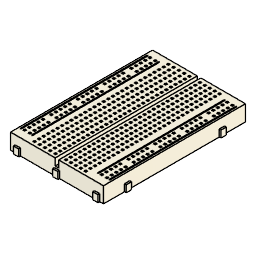
Final Robotic Car (Autodesk Fusion 360 archive; units mm, degrees)
design "Large Breadboard"
part number: 2025-09-23-22-56-39-643
part number: 2025-09-25-13-44-03-592
part number: 2025-09-25-13-51-08-297
part number: 2025-09-25-13-58-47-980
part number: 2025-09-25-14-03-45-841
Autodesk Fusion 360 part; units mm, degrees
(part 1 of 13)
sketch "Sketch1" plane through (0, 0, 0) normal (0, 0, 1) x (1, 0, 0)
  line L0 (26.5, 40.5) -> (-26.5, 40.5)
  line L1 (-26.5, 40.5) -> (-26.5, -40.5)
  line L2 (-26.5, -40.5) -> (26.5, -40.5)
  line L3 (26.5, -40.5) -> (26.5, 40.5)
  line L4 (26.5, 40.5) -> (-26.5, -40.5) construction
  line L5 (-26.5, 40.5) -> (26.5, -40.5) construction
  dimension "d1" = 81
  dimension "d2" = 53
  constraint horizontal L0
  constraint perpendicular L0 L1
  constraint parallel L0 L2
  constraint parallel L1 L3
  constraint coincident L4 origin
  constraint coincident L5 origin
  measures "d1" distance of L0.start L2.end
  measures "d2" distance of L0.start L0.end
extrude "Extrude1" add sketch "Sketch1" along normal blind 9 makes body 1
sketch "Sketch2" plane through (0, 0, 9) normal (0, 0, 1) x (-1, 0, 0)
  line L0 (-26.5, 40.5) -> (-26.5, -40.5)
  line L1 (-26.5, -40.5) -> (26.5, -40.5)
  line L2 (26.5, -40.5) -> (26.5, 40.5)
  line L3 (26.5, 40.5) -> (-26.5, 40.5)
  line L4 (-1, -41) -> (1, -41)
  line L5 (1, -41) -> (1, 41)
  line L6 (1, 41) -> (-1, 41)
  line L7 (-1, 41) -> (-1, -41)
  line L8 (-1, -41) -> (1, 41) construction
  line L9 (1, -41) -> (-1, 41) construction
  dimension "d5" = 2
  dimension "d6" = 82
  constraint horizontal L4
  constraint perpendicular L4 L5
  constraint parallel L4 L6
  constraint parallel L5 L7
  constraint coincident L8 origin
  constraint coincident L9 origin
  measures "d5" distance of L5.end L6.end
  measures "d6" distance of L4.start L6.end
extrude "Extrude2" cut sketch "Sketch2" against normal blind 4 contours L1 L3 L5 L7 bodies 1
sketch "Sketch3" plane through (0, 0, 9) normal (0, 0, 1) x (-1, 0, 0)
  line L0 (-1, -40.5) -> (-1, 40.5)
  line L1 (-1, 40.5) -> (-26.5, 40.5)
  line L2 (-26.5, 40.5) -> (-26.5, -40.5)
  line L3 (-26.5, -40.5) -> (-1, -40.5)
  line L4 (2.5, -37.5) -> (3.5, -37.5)
  line L5 (3.5, -37.5) -> (3.5, -38.5)
  line L6 (3.5, -38.5) -> (2.5, -38.5)
  line L7 (2.5, -38.5) -> (2.5, -37.5)
  line L8 (2.5, -37.5) -> (3.5, -38.5) construction
  line L9 (3.5, -37.5) -> (2.5, -38.5) construction
  line L10 (1, 40.5) -> (1, -40.5)
  line L11 (1, -40.5) -> (26.5, -40.5)
  point P0 (3, -38)
  dimension "d9" = 1
  dimension "d10" = 1
  dimension "d11" = 1.5
  dimension "d12" = 2
  constraint horizontal L4
  constraint perpendicular L4 L5
  constraint parallel L4 L6
  constraint parallel L5 L7
  constraint coincident L8 P0
  constraint coincident L9 P0
  measures "d9" distance of L5.end L6.end
  measures "d10" distance of L4.end L5.end
  measures "d11" distance of L7 L10
  measures "d12" distance of L6 L11
extrude "Extrude3" cut sketch "Sketch3" against normal blind 1 contours L4 L5 L6 L7 bodies 1
pattern_linear "R-Pattern1" count 5 spacing 3 along (-1, 0, 0) count 30 spacing 2.63 along (0, -1, 0) of "Extrude3"
sketch "Sketch4" plane through (0, 0, 9) normal (0, 0, 1) x (-1, 0, 0)
  line L0 (-1, -40.5) -> (-1, 40.5)
  line L1 (-1, 40.5) -> (-26.5, 40.5)
  line L2 (-26.5, 40.5) -> (-26.5, -40.5)
  line L3 (-26.5, -40.5) -> (-1, -40.5)
  line L4 (-3.5, -37.5) -> (-2.5, -37.5)
  line L5 (-2.5, -37.5) -> (-2.5, -38.5)
  line L6 (-2.5, -38.5) -> (-3.5, -38.5)
  line L7 (-3.5, -38.5) -> (-3.5, -37.5)
  line L8 (-3.5, -37.5) -> (-2.5, -38.5) construction
  line L9 (-2.5, -37.5) -> (-3.5, -38.5) construction
  point P0 (-3, -38)
  dimension "d19" = 1
  dimension "d20" = 1
  dimension "d21" = 2
  dimension "d22" = 1.5
  constraint horizontal L4
  constraint perpendicular L4 L5
  constraint parallel L4 L6
  constraint parallel L5 L7
  constraint coincident L8 P0
  constraint coincident L9 P0
  measures "d19" distance of L5.end L6.end
  measures "d20" distance of L4.start L6.end
  measures "d21" distance of L3 L6
  measures "d22" distance of L0 L5
extrude "Extrude4" cut sketch "Sketch4" against normal blind 1 contours L4 L5 L6 L7 bodies 1
sketch "Sketch5" plane through (0, 0, 9) normal (0, 0, 1) x (-1, 0, 0)
  line L0 (15.5, 38.77) -> (15.5, 37.77)
  line L1 (15.5, 37.77) -> (14.5, 37.77)
  line L2 (14.5, 37.77) -> (14.5, 38.77)
  line L3 (14.5, 38.77) -> (15.5, 38.77)
  line L4 (12.5, 38.77) -> (12.5, 37.77)
  line L5 (12.5, 37.77) -> (11.5, 37.77)
  line L6 (11.5, 37.77) -> (11.5, 38.77)
  line L7 (11.5, 38.77) -> (12.5, 38.77)
  line L8 (9.5, 38.77) -> (9.5, 37.77)
  line L9 (9.5, 37.77) -> (8.5, 37.77)
  line L10 (8.5, 37.77) -> (8.5, 38.77)
  line L11 (8.5, 38.77) -> (9.5, 38.77)
  line L12 (6.5, 38.77) -> (6.5, 37.77)
  line L13 (6.5, 37.77) -> (5.5, 37.77)
  line L14 (5.5, 37.77) -> (5.5, 38.77)
  line L15 (5.5, 38.77) -> (6.5, 38.77)
  line L16 (3.5, 38.77) -> (3.5, 37.77)
  line L17 (3.5, 37.77) -> (2.5, 37.77)
  line L18 (2.5, 37.77) -> (2.5, 38.77)
  line L19 (2.5, 38.77) -> (3.5, 38.77)
  line L20 (15.5, 36.14) -> (15.5, 35.14)
  line L21 (15.5, 35.14) -> (14.5, 35.14)
  line L22 (14.5, 35.14) -> (14.5, 36.14)
  line L23 (14.5, 36.14) -> (15.5, 36.14)
  line L24 (12.5, 36.14) -> (12.5, 35.14)
  line L25 (12.5, 35.14) -> (11.5, 35.14)
  line L26 (11.5, 35.14) -> (11.5, 36.14)
  line L27 (11.5, 36.14) -> (12.5, 36.14)
  line L28 (9.5, 36.14) -> (9.5, 35.14)
  line L29 (9.5, 35.14) -> (8.5, 35.14)
  line L30 (8.5, 35.14) -> (8.5, 36.14)
  line L31 (8.5, 36.14) -> (9.5, 36.14)
  line L32 (6.5, 36.14) -> (6.5, 35.14)
  line L33 (6.5, 35.14) -> (5.5, 35.14)
  line L34 (5.5, 35.14) -> (5.5, 36.14)
  line L35 (5.5, 36.14) -> (6.5, 36.14)
  line L36 (3.5, 36.14) -> (3.5, 35.14)
  line L37 (3.5, 35.14) -> (2.5, 35.14)
  line L38 (2.5, 35.14) -> (2.5, 36.14)
  line L39 (2.5, 36.14) -> (3.5, 36.14)
  line L40 (15.5, 33.51) -> (15.5, 32.51)
  line L41 (15.5, 32.51) -> (14.5, 32.51)
  line L42 (14.5, 32.51) -> (14.5, 33.51)
  line L43 (14.5, 33.51) -> (15.5, 33.51)
  line L44 (12.5, 33.51) -> (12.5, 32.51)
  line L45 (12.5, 32.51) -> (11.5, 32.51)
  line L46 (11.5, 32.51) -> (11.5, 33.51)
  line L47 (11.5, 33.51) -> (12.5, 33.51)
  line L48 (9.5, 33.51) -> (9.5, 32.51)
  line L49 (9.5, 32.51) -> (8.5, 32.51)
  line L50 (8.5, 32.51) -> (8.5, 33.51)
  line L51 (8.5, 33.51) -> (9.5, 33.51)
  line L52 (6.5, 33.51) -> (6.5, 32.51)
  line L53 (6.5, 32.51) -> (5.5, 32.51)
  line L54 (5.5, 32.51) -> (5.5, 33.51)
  line L55 (5.5, 33.51) -> (6.5, 33.51)
  line L56 (3.5, 33.51) -> (3.5, 32.51)
  line L57 (3.5, 32.51) -> (2.5, 32.51)
  line L58 (2.5, 32.51) -> (2.5, 33.51)
  line L59 (2.5, 33.51) -> (3.5, 33.51)
  line L60 (15.5, 30.88) -> (15.5, 29.88)
  line L61 (15.5, 29.88) -> (14.5, 29.88)
  line L62 (14.5, 29.88) -> (14.5, 30.88)
  line L63 (14.5, 30.88) -> (15.5, 30.88)
  line L64 (12.5, 30.88) -> (12.5, 29.88)
  line L65 (12.5, 29.88) -> (11.5, 29.88)
  line L66 (11.5, 29.88) -> (11.5, 30.88)
  line L67 (11.5, 30.88) -> (12.5, 30.88)
  line L68 (9.5, 30.88) -> (9.5, 29.88)
  line L69 (9.5, 29.88) -> (8.5, 29.88)
  line L70 (8.5, 29.88) -> (8.5, 30.88)
  line L71 (8.5, 30.88) -> (9.5, 30.88)
  line L72 (6.5, 30.88) -> (6.5, 29.88)
  line L73 (6.5, 29.88) -> (5.5, 29.88)
  line L74 (5.5, 29.88) -> (5.5, 30.88)
  line L75 (5.5, 30.88) -> (6.5, 30.88)
  line L76 (3.5, 30.88) -> (3.5, 29.88)
  line L77 (3.5, 29.88) -> (2.5, 29.88)
  line L78 (2.5, 29.88) -> (2.5, 30.88)
  line L79 (2.5, 30.88) -> (3.5, 30.88)
  line L80 (15.5, 28.25) -> (15.5, 27.25)
  line L81 (15.5, 27.25) -> (14.5, 27.25)
  line L82 (14.5, 27.25) -> (14.5, 28.25)
  line L83 (14.5, 28.25) -> (15.5, 28.25)
  line L84 (12.5, 28.25) -> (12.5, 27.25)
  line L85 (12.5, 27.25) -> (11.5, 27.25)
  line L86 (11.5, 27.25) -> (11.5, 28.25)
  line L87 (11.5, 28.25) -> (12.5, 28.25)
  line L88 (9.5, 28.25) -> (9.5, 27.25)
  line L89 (9.5, 27.25) -> (8.5, 27.25)
  line L90 (8.5, 27.25) -> (8.5, 28.25)
  line L91 (8.5, 28.25) -> (9.5, 28.25)
  line L92 (6.5, 28.25) -> (6.5, 27.25)
  line L93 (6.5, 27.25) -> (5.5, 27.25)
  line L94 (5.5, 27.25) -> (5.5, 28.25)
  line L95 (5.5, 28.25) -> (6.5, 28.25)
  line L96 (3.5, 28.25) -> (3.5, 27.25)
  line L97 (3.5, 27.25) -> (2.5, 27.25)
  line L98 (2.5, 27.25) -> (2.5, 28.25)
  line L99 (2.5, 28.25) -> (3.5, 28.25)
  line L100 (15.5, 25.62) -> (15.5, 24.62)
  line L101 (15.5, 24.62) -> (14.5, 24.62)
  line L102 (14.5, 24.62) -> (14.5, 25.62)
  line L103 (14.5, 25.62) -> (15.5, 25.62)
  line L104 (12.5, 25.62) -> (12.5, 24.62)
  line L105 (12.5, 24.62) -> (11.5, 24.62)
  line L106 (11.5, 24.62) -> (11.5, 25.62)
  line L107 (11.5, 25.62) -> (12.5, 25.62)
  line L108 (9.5, 25.62) -> (9.5, 24.62)
  line L109 (9.5, 24.62) -> (8.5, 24.62)
  line L110 (8.5, 24.62) -> (8.5, 25.62)
  line L111 (8.5, 25.62) -> (9.5, 25.62)
  line L112 (6.5, 25.62) -> (6.5, 24.62)
  line L113 (6.5, 24.62) -> (5.5, 24.62)
  line L114 (5.5, 24.62) -> (5.5, 25.62)
  line L115 (5.5, 25.62) -> (6.5, 25.62)
  line L116 (3.5, 25.62) -> (3.5, 24.62)
  line L117 (3.5, 24.62) -> (2.5, 24.62)
  line L118 (2.5, 24.62) -> (2.5, 25.62)
  line L119 (2.5, 25.62) -> (3.5, 25.62)
  line L120 (15.5, 22.99) -> (15.5, 21.99)
  line L121 (15.5, 21.99) -> (14.5, 21.99)
  line L122 (14.5, 21.99) -> (14.5, 22.99)
  line L123 (14.5, 22.99) -> (15.5, 22.99)
  line L124 (12.5, 22.99) -> (12.5, 21.99)
  line L125 (12.5, 21.99) -> (11.5, 21.99)
  line L126 (11.5, 21.99) -> (11.5, 22.99)
  line L127 (11.5, 22.99) -> (12.5, 22.99)
  line L128 (9.5, 22.99) -> (9.5, 21.99)
  line L129 (9.5, 21.99) -> (8.5, 21.99)
  line L130 (8.5, 21.99) -> (8.5, 22.99)
  line L131 (8.5, 22.99) -> (9.5, 22.99)
  line L132 (6.5, 22.99) -> (6.5, 21.99)
  line L133 (6.5, 21.99) -> (5.5, 21.99)
  line L134 (5.5, 21.99) -> (5.5, 22.99)
  line L135 (5.5, 22.99) -> (6.5, 22.99)
  line L136 (3.5, 22.99) -> (3.5, 21.99)
  line L137 (3.5, 21.99) -> (2.5, 21.99)
  line L138 (2.5, 21.99) -> (2.5, 22.99)
  line L139 (2.5, 22.99) -> (3.5, 22.99)
  line L140 (15.5, 20.36) -> (15.5, 19.36)
  line L141 (15.5, 19.36) -> (14.5, 19.36)
  line L142 (14.5, 19.36) -> (14.5, 20.36)
  line L143 (14.5, 20.36) -> (15.5, 20.36)
  line L144 (12.5, 20.36) -> (12.5, 19.36)
  line L145 (12.5, 19.36) -> (11.5, 19.36)
  line L146 (11.5, 19.36) -> (11.5, 20.36)
  line L147 (11.5, 20.36) -> (12.5, 20.36)
  line L148 (9.5, 20.36) -> (9.5, 19.36)
  line L149 (9.5, 19.36) -> (8.5, 19.36)
  line L150 (8.5, 19.36) -> (8.5, 20.36)
  line L151 (8.5, 20.36) -> (9.5, 20.36)
  line L152 (6.5, 20.36) -> (6.5, 19.36)
  line L153 (6.5, 19.36) -> (5.5, 19.36)
  line L154 (5.5, 19.36) -> (5.5, 20.36)
  line L155 (5.5, 20.36) -> (6.5, 20.36)
  line L156 (3.5, 20.36) -> (3.5, 19.36)
  line L157 (3.5, 19.36) -> (2.5, 19.36)
  line L158 (2.5, 19.36) -> (2.5, 20.36)
  line L159 (2.5, 20.36) -> (3.5, 20.36)
  line L160 (15.5, 17.73) -> (15.5, 16.73)
  line L161 (15.5, 16.73) -> (14.5, 16.73)
  line L162 (14.5, 16.73) -> (14.5, 17.73)
  line L163 (14.5, 17.73) -> (15.5, 17.73)
  line L164 (12.5, 17.73) -> (12.5, 16.73)
  line L165 (12.5, 16.73) -> (11.5, 16.73)
  line L166 (11.5, 16.73) -> (11.5, 17.73)
  line L167 (11.5, 17.73) -> (12.5, 17.73)
  line L168 (9.5, 17.73) -> (9.5, 16.73)
  line L169 (9.5, 16.73) -> (8.5, 16.73)
  line L170 (8.5, 16.73) -> (8.5, 17.73)
  line L171 (8.5, 17.73) -> (9.5, 17.73)
  line L172 (6.5, 17.73) -> (6.5, 16.73)
  line L173 (6.5, 16.73) -> (5.5, 16.73)
  line L174 (5.5, 16.73) -> (5.5, 17.73)
  line L175 (5.5, 17.73) -> (6.5, 17.73)
  line L176 (3.5, 17.73) -> (3.5, 16.73)
  line L177 (3.5, 16.73) -> (2.5, 16.73)
  line L178 (2.5, 16.73) -> (2.5, 17.73)
  line L179 (2.5, 17.73) -> (3.5, 17.73)
  line L180 (15.5, 15.1) -> (15.5, 14.1)
  line L181 (15.5, 14.1) -> (14.5, 14.1)
  line L182 (14.5, 14.1) -> (14.5, 15.1)
  line L183 (14.5, 15.1) -> (15.5, 15.1)
  line L184 (12.5, 15.1) -> (12.5, 14.1)
  line L185 (12.5, 14.1) -> (11.5, 14.1)
  line L186 (11.5, 14.1) -> (11.5, 15.1)
  line L187 (11.5, 15.1) -> (12.5, 15.1)
  line L188 (9.5, 15.1) -> (9.5, 14.1)
  line L189 (9.5, 14.1) -> (8.5, 14.1)
  line L190 (8.5, 14.1) -> (8.5, 15.1)
  line L191 (8.5, 15.1) -> (9.5, 15.1)
  line L192 (6.5, 15.1) -> (6.5, 14.1)
  line L193 (6.5, 14.1) -> (5.5, 14.1)
  line L194 (5.5, 14.1) -> (5.5, 15.1)
  line L195 (5.5, 15.1) -> (6.5, 15.1)
  line L196 (3.5, 15.1) -> (3.5, 14.1)
  line L197 (3.5, 14.1) -> (2.5, 14.1)
  line L198 (2.5, 14.1) -> (2.5, 15.1)
  line L199 (2.5, 15.1) -> (3.5, 15.1)
  line L200 (15.5, 12.47) -> (15.5, 11.47)
  line L201 (15.5, 11.47) -> (14.5, 11.47)
  line L202 (14.5, 11.47) -> (14.5, 12.47)
  line L203 (14.5, 12.47) -> (15.5, 12.47)
  line L204 (12.5, 12.47) -> (12.5, 11.47)
  line L205 (12.5, 11.47) -> (11.5, 11.47)
  line L206 (11.5, 11.47) -> (11.5, 12.47)
  line L207 (11.5, 12.47) -> (12.5, 12.47)
  line L208 (9.5, 12.47) -> (9.5, 11.47)
  line L209 (9.5, 11.47) -> (8.5, 11.47)
  line L210 (8.5, 11.47) -> (8.5, 12.47)
  line L211 (8.5, 12.47) -> (9.5, 12.47)
  line L212 (6.5, 12.47) -> (6.5, 11.47)
  line L213 (6.5, 11.47) -> (5.5, 11.47)
  line L214 (5.5, 11.47) -> (5.5, 12.47)
  line L215 (5.5, 12.47) -> (6.5, 12.47)
  line L216 (3.5, 12.47) -> (3.5, 11.47)
  line L217 (3.5, 11.47) -> (2.5, 11.47)
  line L218 (2.5, 11.47) -> (2.5, 12.47)
  line L219 (2.5, 12.47) -> (3.5, 12.47)
  line L220 (15.5, 9.84) -> (15.5, 8.84)
  line L221 (15.5, 8.84) -> (14.5, 8.84)
  line L222 (14.5, 8.84) -> (14.5, 9.84)
  line L223 (14.5, 9.84) -> (15.5, 9.84)
  line L224 (12.5, 9.84) -> (12.5, 8.84)
  line L225 (12.5, 8.84) -> (11.5, 8.84)
  line L226 (11.5, 8.84) -> (11.5, 9.84)
  line L227 (11.5, 9.84) -> (12.5, 9.84)
  line L228 (9.5, 9.84) -> (9.5, 8.84)
  line L229 (9.5, 8.84) -> (8.5, 8.84)
  line L230 (8.5, 8.84) -> (8.5, 9.84)
  line L231 (8.5, 9.84) -> (9.5, 9.84)
  line L232 (6.5, 9.84) -> (6.5, 8.84)
  line L233 (6.5, 8.84) -> (5.5, 8.84)
  line L234 (5.5, 8.84) -> (5.5, 9.84)
  line L235 (5.5, 9.84) -> (6.5, 9.84)
  line L236 (3.5, 9.84) -> (3.5, 8.84)
  line L237 (3.5, 8.84) -> (2.5, 8.84)
  line L238 (2.5, 8.84) -> (2.5, 9.84)
  line L239 (2.5, 9.84) -> (3.5, 9.84)
  line L240 (15.5, 7.21) -> (15.5, 6.21)
  line L241 (15.5, 6.21) -> (14.5, 6.21)
  line L242 (14.5, 6.21) -> (14.5, 7.21)
  line L243 (14.5, 7.21) -> (15.5, 7.21)
  line L244 (12.5, 7.21) -> (12.5, 6.21)
  line L245 (12.5, 6.21) -> (11.5, 6.21)
  line L246 (11.5, 6.21) -> (11.5, 7.21)
  line L247 (11.5, 7.21) -> (12.5, 7.21)
  line L248 (9.5, 7.21) -> (9.5, 6.21)
  line L249 (9.5, 6.21) -> (8.5, 6.21)
  line L250 (8.5, 6.21) -> (8.5, 7.21)
  line L251 (8.5, 7.21) -> (9.5, 7.21)
  line L252 (6.5, 7.21) -> (6.5, 6.21)
  line L253 (6.5, 6.21) -> (5.5, 6.21)
  line L254 (5.5, 6.21) -> (5.5, 7.21)
  line L255 (5.5, 7.21) -> (6.5, 7.21)
  line L256 (3.5, 7.21) -> (3.5, 6.21)
  line L257 (3.5, 6.21) -> (2.5, 6.21)
  line L258 (2.5, 6.21) -> (2.5, 7.21)
  line L259 (2.5, 7.21) -> (3.5, 7.21)
  line L260 (15.5, 4.58) -> (15.5, 3.58)
  line L261 (15.5, 3.58) -> (14.5, 3.58)
  line L262 (14.5, 3.58) -> (14.5, 4.58)
  line L263 (14.5, 4.58) -> (15.5, 4.58)
  line L264 (12.5, 4.58) -> (12.5, 3.58)
  line L265 (12.5, 3.58) -> (11.5, 3.58)
  line L266 (11.5, 3.58) -> (11.5, 4.58)
  line L267 (11.5, 4.58) -> (12.5, 4.58)
  line L268 (9.5, 4.58) -> (9.5, 3.58)
  line L269 (9.5, 3.58) -> (8.5, 3.58)
  line L270 (8.5, 3.58) -> (8.5, 4.58)
  line L271 (8.5, 4.58) -> (9.5, 4.58)
  line L272 (6.5, 4.58) -> (6.5, 3.58)
  line L273 (6.5, 3.58) -> (5.5, 3.58)
  line L274 (5.5, 3.58) -> (5.5, 4.58)
  line L275 (5.5, 4.58) -> (6.5, 4.58)
  line L276 (3.5, 4.58) -> (3.5, 3.58)
  line L277 (3.5, 3.58) -> (2.5, 3.58)
  line L278 (2.5, 3.58) -> (2.5, 4.58)
  line L279 (2.5, 4.58) -> (3.5, 4.58)
  line L280 (15.5, 1.95) -> (15.5, 0.95)
  line L281 (15.5, 0.95) -> (14.5, 0.95)
  line L282 (14.5, 0.95) -> (14.5, 1.95)
  line L283 (14.5, 1.95) -> (15.5, 1.95)
  line L284 (12.5, 1.95) -> (12.5, 0.95)
  line L285 (12.5, 0.95) -> (11.5, 0.95)
  line L286 (11.5, 0.95) -> (11.5, 1.95)
  line L287 (11.5, 1.95) -> (12.5, 1.95)
  line L288 (9.5, 1.95) -> (9.5, 0.95)
  line L289 (9.5, 0.95) -> (8.5, 0.95)
  line L290 (8.5, 0.95) -> (8.5, 1.95)
  line L291 (8.5, 1.95) -> (9.5, 1.95)
  line L292 (6.5, 1.95) -> (6.5, 0.95)
  line L293 (6.5, 0.95) -> (5.5, 0.95)
  line L294 (5.5, 0.95) -> (5.5, 1.95)
  line L295 (5.5, 1.95) -> (6.5, 1.95)
  line L296 (3.5, 1.95) -> (3.5, 0.95)
  line L297 (3.5, 0.95) -> (2.5, 0.95)
  line L298 (2.5, 0.95) -> (2.5, 1.95)
  line L299 (2.5, 1.95) -> (3.5, 1.95)
  line L300 (15.5, -0.68) -> (15.5, -1.68)
  line L301 (15.5, -1.68) -> (14.5, -1.68)
  line L302 (14.5, -1.68) -> (14.5, -0.68)
  line L303 (14.5, -0.68) -> (15.5, -0.68)
  line L304 (12.5, -0.68) -> (12.5, -1.68)
  line L305 (12.5, -1.68) -> (11.5, -1.68)
  line L306 (11.5, -1.68) -> (11.5, -0.68)
  line L307 (11.5, -0.68) -> (12.5, -0.68)
  line L308 (9.5, -0.68) -> (9.5, -1.68)
  line L309 (9.5, -1.68) -> (8.5, -1.68)
  line L310 (8.5, -1.68) -> (8.5, -0.68)
  line L311 (8.5, -0.68) -> (9.5, -0.68)
  line L312 (6.5, -0.68) -> (6.5, -1.68)
  line L313 (6.5, -1.68) -> (5.5, -1.68)
  line L314 (5.5, -1.68) -> (5.5, -0.68)
  line L315 (5.5, -0.68) -> (6.5, -0.68)
  line L316 (3.5, -0.68) -> (3.5, -1.68)
  line L317 (3.5, -1.68) -> (2.5, -1.68)
  line L318 (2.5, -1.68) -> (2.5, -0.68)
  line L319 (2.5, -0.68) -> (3.5, -0.68)
  line L320 (15.5, -3.31) -> (15.5, -4.31)
  line L321 (15.5, -4.31) -> (14.5, -4.31)
  line L322 (14.5, -4.31) -> (14.5, -3.31)
  line L323 (14.5, -3.31) -> (15.5, -3.31)
  line L324 (12.5, -3.31) -> (12.5, -4.31)
  line L325 (12.5, -4.31) -> (11.5, -4.31)
  line L326 (11.5, -4.31) -> (11.5, -3.31)
  line L327 (11.5, -3.31) -> (12.5, -3.31)
  line L328 (9.5, -3.31) -> (9.5, -4.31)
  line L329 (9.5, -4.31) -> (8.5, -4.31)
  line L330 (8.5, -4.31) -> (8.5, -3.31)
  line L331 (8.5, -3.31) -> (9.5, -3.31)
  line L332 (6.5, -3.31) -> (6.5, -4.31)
  line L333 (6.5, -4.31) -> (5.5, -4.31)
  line L334 (5.5, -4.31) -> (5.5, -3.31)
  line L335 (5.5, -3.31) -> (6.5, -3.31)
  line L336 (3.5, -3.31) -> (3.5, -4.31)
  line L337 (3.5, -4.31) -> (2.5, -4.31)
  line L338 (2.5, -4.31) -> (2.5, -3.31)
  line L339 (2.5, -3.31) -> (3.5, -3.31)
  line L340 (15.5, -5.94) -> (15.5, -6.94)
  line L341 (15.5, -6.94) -> (14.5, -6.94)
  line L342 (14.5, -6.94) -> (14.5, -5.94)
  line L343 (14.5, -5.94) -> (15.5, -5.94)
  line L344 (12.5, -5.94) -> (12.5, -6.94)
  line L345 (12.5, -6.94) -> (11.5, -6.94)
  line L346 (11.5, -6.94) -> (11.5, -5.94)
  line L347 (11.5, -5.94) -> (12.5, -5.94)
  line L348 (9.5, -5.94) -> (9.5, -6.94)
  line L349 (9.5, -6.94) -> (8.5, -6.94)
  line L350 (8.5, -6.94) -> (8.5, -5.94)
  line L351 (8.5, -5.94) -> (9.5, -5.94)
  line L352 (6.5, -5.94) -> (6.5, -6.94)
  line L353 (6.5, -6.94) -> (5.5, -6.94)
  line L354 (5.5, -6.94) -> (5.5, -5.94)
  line L355 (5.5, -5.94) -> (6.5, -5.94)
  line L356 (3.5, -5.94) -> (3.5, -6.94)
  line L357 (3.5, -6.94) -> (2.5, -6.94)
  line L358 (2.5, -6.94) -> (2.5, -5.94)
  line L359 (2.5, -5.94) -> (3.5, -5.94)
  line L360 (15.5, -8.57) -> (15.5, -9.57)
  line L361 (15.5, -9.57) -> (14.5, -9.57)
  line L362 (14.5, -9.57) -> (14.5, -8.57)
  line L363 (14.5, -8.57) -> (15.5, -8.57)
  line L364 (12.5, -8.57) -> (12.5, -9.57)
  line L365 (12.5, -9.57) -> (11.5, -9.57)
  line L366 (11.5, -9.57) -> (11.5, -8.57)
  line L367 (11.5, -8.57) -> (12.5, -8.57)
  line L368 (9.5, -8.57) -> (9.5, -9.57)
  line L369 (9.5, -9.57) -> (8.5, -9.57)
  line L370 (8.5, -9.57) -> (8.5, -8.57)
  line L371 (8.5, -8.57) -> (9.5, -8.57)
  line L372 (6.5, -8.57) -> (6.5, -9.57)
  line L373 (6.5, -9.57) -> (5.5, -9.57)
  line L374 (5.5, -9.57) -> (5.5, -8.57)
  line L375 (5.5, -8.57) -> (6.5, -8.57)
  line L376 (3.5, -8.57) -> (3.5, -9.57)
  line L377 (3.5, -9.57) -> (2.5, -9.57)
  line L378 (2.5, -9.57) -> (2.5, -8.57)
  line L379 (2.5, -8.57) -> (3.5, -8.57)
  line L380 (15.5, -11.2) -> (15.5, -12.2)
  line L381 (15.5, -12.2) -> (14.5, -12.2)
  line L382 (14.5, -12.2) -> (14.5, -11.2)
  line L383 (14.5, -11.2) -> (15.5, -11.2)
  line L384 (12.5, -11.2) -> (12.5, -12.2)
  line L385 (12.5, -12.2) -> (11.5, -12.2)
  line L386 (11.5, -12.2) -> (11.5, -11.2)
  line L387 (11.5, -11.2) -> (12.5, -11.2)
  line L388 (9.5, -11.2) -> (9.5, -12.2)
  line L389 (9.5, -12.2) -> (8.5, -12.2)
  line L390 (8.5, -12.2) -> (8.5, -11.2)
  line L391 (8.5, -11.2) -> (9.5, -11.2)
  line L392 (6.5, -11.2) -> (6.5, -12.2)
  line L393 (6.5, -12.2) -> (5.5, -12.2)
  line L394 (5.5, -12.2) -> (5.5, -11.2)
  line L395 (5.5, -11.2) -> (6.5, -11.2)
  line L396 (3.5, -11.2) -> (3.5, -12.2)
  line L397 (3.5, -12.2) -> (2.5, -12.2)
  line L398 (2.5, -12.2) -> (2.5, -11.2)
  line L399 (2.5, -11.2) -> (3.5, -11.2)
  line L400 (15.5, -13.83) -> (15.5, -14.83)
  line L401 (15.5, -14.83) -> (14.5, -14.83)
  line L402 (14.5, -14.83) -> (14.5, -13.83)
  line L403 (14.5, -13.83) -> (15.5, -13.83)
  line L404 (12.5, -13.83) -> (12.5, -14.83)
  line L405 (12.5, -14.83) -> (11.5, -14.83)
  line L406 (11.5, -14.83) -> (11.5, -13.83)
  line L407 (11.5, -13.83) -> (12.5, -13.83)
  line L408 (9.5, -13.83) -> (9.5, -14.83)
  line L409 (9.5, -14.83) -> (8.5, -14.83)
  line L410 (8.5, -14.83) -> (8.5, -13.83)
  line L411 (8.5, -13.83) -> (9.5, -13.83)
  line L412 (6.5, -13.83) -> (6.5, -14.83)
  line L413 (6.5, -14.83) -> (5.5, -14.83)
  line L414 (5.5, -14.83) -> (5.5, -13.83)
  line L415 (5.5, -13.83) -> (6.5, -13.83)
  line L416 (3.5, -13.83) -> (3.5, -14.83)
  line L417 (3.5, -14.83) -> (2.5, -14.83)
  line L418 (2.5, -14.83) -> (2.5, -13.83)
  line L419 (2.5, -13.83) -> (3.5, -13.83)
  line L420 (15.5, -16.46) -> (15.5, -17.46)
  line L421 (15.5, -17.46) -> (14.5, -17.46)
  line L422 (14.5, -17.46) -> (14.5, -16.46)
  line L423 (14.5, -16.46) -> (15.5, -16.46)
  line L424 (12.5, -16.46) -> (12.5, -17.46)
  line L425 (12.5, -17.46) -> (11.5, -17.46)
  line L426 (11.5, -17.46) -> (11.5, -16.46)
  line L427 (11.5, -16.46) -> (12.5, -16.46)
  line L428 (9.5, -16.46) -> (9.5, -17.46)
  line L429 (9.5, -17.46) -> (8.5, -17.46)
  line L430 (8.5, -17.46) -> (8.5, -16.46)
  line L431 (8.5, -16.46) -> (9.5, -16.46)
  line L432 (6.5, -16.46) -> (6.5, -17.46)
  line L433 (6.5, -17.46) -> (5.5, -17.46)
  line L434 (5.5, -17.46) -> (5.5, -16.46)
  line L435 (5.5, -16.46) -> (6.5, -16.46)
  line L436 (3.5, -16.46) -> (3.5, -17.46)
  line L437 (3.5, -17.46) -> (2.5, -17.46)
  line L438 (2.5, -17.46) -> (2.5, -16.46)
  line L439 (2.5, -16.46) -> (3.5, -16.46)
  line L440 (15.5, -19.09) -> (15.5, -20.09)
  line L441 (15.5, -20.09) -> (14.5, -20.09)
  line L442 (14.5, -20.09) -> (14.5, -19.09)
  line L443 (14.5, -19.09) -> (15.5, -19.09)
  line L444 (12.5, -19.09) -> (12.5, -20.09)
  line L445 (12.5, -20.09) -> (11.5, -20.09)
  line L446 (11.5, -20.09) -> (11.5, -19.09)
  line L447 (11.5, -19.09) -> (12.5, -19.09)
  line L448 (9.5, -19.09) -> (9.5, -20.09)
  line L449 (9.5, -20.09) -> (8.5, -20.09)
  line L450 (8.5, -20.09) -> (8.5, -19.09)
  line L451 (8.5, -19.09) -> (9.5, -19.09)
  line L452 (6.5, -19.09) -> (6.5, -20.09)
  line L453 (6.5, -20.09) -> (5.5, -20.09)
  line L454 (5.5, -20.09) -> (5.5, -19.09)
  line L455 (5.5, -19.09) -> (6.5, -19.09)
  line L456 (3.5, -19.09) -> (3.5, -20.09)
  line L457 (3.5, -20.09) -> (2.5, -20.09)
  line L458 (2.5, -20.09) -> (2.5, -19.09)
  line L459 (2.5, -19.09) -> (3.5, -19.09)
  line L460 (15.5, -21.72) -> (15.5, -22.72)
  line L461 (15.5, -22.72) -> (14.5, -22.72)
  line L462 (14.5, -22.72) -> (14.5, -21.72)
  line L463 (14.5, -21.72) -> (15.5, -21.72)
  line L464 (12.5, -21.72) -> (12.5, -22.72)
  line L465 (12.5, -22.72) -> (11.5, -22.72)
  line L466 (11.5, -22.72) -> (11.5, -21.72)
  line L467 (11.5, -21.72) -> (12.5, -21.72)
  line L468 (9.5, -21.72) -> (9.5, -22.72)
  line L469 (9.5, -22.72) -> (8.5, -22.72)
  line L470 (8.5, -22.72) -> (8.5, -21.72)
  line L471 (8.5, -21.72) -> (9.5, -21.72)
  line L472 (6.5, -21.72) -> (6.5, -22.72)
  line L473 (6.5, -22.72) -> (5.5, -22.72)
  line L474 (5.5, -22.72) -> (5.5, -21.72)
  line L475 (5.5, -21.72) -> (6.5, -21.72)
  line L476 (3.5, -21.72) -> (3.5, -22.72)
  line L477 (3.5, -22.72) -> (2.5, -22.72)
  line L478 (2.5, -22.72) -> (2.5, -21.72)
  line L479 (2.5, -21.72) -> (3.5, -21.72)
  line L480 (15.5, -24.35) -> (15.5, -25.35)
  line L481 (15.5, -25.35) -> (14.5, -25.35)
  line L482 (14.5, -25.35) -> (14.5, -24.35)
  line L483 (14.5, -24.35) -> (15.5, -24.35)
  line L484 (12.5, -24.35) -> (12.5, -25.35)
  line L485 (12.5, -25.35) -> (11.5, -25.35)
  line L486 (11.5, -25.35) -> (11.5, -24.35)
  line L487 (11.5, -24.35) -> (12.5, -24.35)
  line L488 (9.5, -24.35) -> (9.5, -25.35)
  line L489 (9.5, -25.35) -> (8.5, -25.35)
  line L490 (8.5, -25.35) -> (8.5, -24.35)
  line L491 (8.5, -24.35) -> (9.5, -24.35)
  line L492 (6.5, -24.35) -> (6.5, -25.35)
  line L493 (6.5, -25.35) -> (5.5, -25.35)
  line L494 (5.5, -25.35) -> (5.5, -24.35)
  line L495 (5.5, -24.35) -> (6.5, -24.35)
  line L496 (3.5, -24.35) -> (3.5, -25.35)
  line L497 (3.5, -25.35) -> (2.5, -25.35)
  line L498 (2.5, -25.35) -> (2.5, -24.35)
  line L499 (2.5, -24.35) -> (3.5, -24.35)
  line L500 (15.5, -26.98) -> (15.5, -27.98)
  line L501 (15.5, -27.98) -> (14.5, -27.98)
  line L502 (14.5, -27.98) -> (14.5, -26.98)
  line L503 (14.5, -26.98) -> (15.5, -26.98)
  line L504 (12.5, -26.98) -> (12.5, -27.98)
  line L505 (12.5, -27.98) -> (11.5, -27.98)
  line L506 (11.5, -27.98) -> (11.5, -26.98)
  line L507 (11.5, -26.98) -> (12.5, -26.98)
  line L508 (9.5, -26.98) -> (9.5, -27.98)
  line L509 (9.5, -27.98) -> (8.5, -27.98)
  line L510 (8.5, -27.98) -> (8.5, -26.98)
  line L511 (8.5, -26.98) -> (9.5, -26.98)
  line L512 (6.5, -26.98) -> (6.5, -27.98)
  line L513 (6.5, -27.98) -> (5.5, -27.98)
  line L514 (5.5, -27.98) -> (5.5, -26.98)
  line L515 (5.5, -26.98) -> (6.5, -26.98)
  line L516 (3.5, -26.98) -> (3.5, -27.98)
  line L517 (3.5, -27.98) -> (2.5, -27.98)
  line L518 (2.5, -27.98) -> (2.5, -26.98)
  line L519 (2.5, -26.98) -> (3.5, -26.98)
  line L520 (15.5, -29.61) -> (15.5, -30.61)
  line L521 (15.5, -30.61) -> (14.5, -30.61)
  line L522 (14.5, -30.61) -> (14.5, -29.61)
  line L523 (14.5, -29.61) -> (15.5, -29.61)
  line L524 (12.5, -29.61) -> (12.5, -30.61)
  line L525 (12.5, -30.61) -> (11.5, -30.61)
  line L526 (11.5, -30.61) -> (11.5, -29.61)
  line L527 (11.5, -29.61) -> (12.5, -29.61)
  line L528 (9.5, -29.61) -> (9.5, -30.61)
  line L529 (9.5, -30.61) -> (8.5, -30.61)
  line L530 (8.5, -30.61) -> (8.5, -29.61)
  line L531 (8.5, -29.61) -> (9.5, -29.61)
  line L532 (6.5, -29.61) -> (6.5, -30.61)
  line L533 (6.5, -30.61) -> (5.5, -30.61)
  line L534 (5.5, -30.61) -> (5.5, -29.61)
  line L535 (5.5, -29.61) -> (6.5, -29.61)
  line L536 (3.5, -29.61) -> (3.5, -30.61)
  line L537 (3.5, -30.61) -> (2.5, -30.61)
  line L538 (2.5, -30.61) -> (2.5, -29.61)
  line L539 (2.5, -29.61) -> (3.5, -29.61)
  line L540 (15.5, -32.24) -> (15.5, -33.24)
  line L541 (15.5, -33.24) -> (14.5, -33.24)
  line L542 (14.5, -33.24) -> (14.5, -32.24)
  line L543 (14.5, -32.24) -> (15.5, -32.24)
  line L544 (12.5, -32.24) -> (12.5, -33.24)
  line L545 (12.5, -33.24) -> (11.5, -33.24)
  line L546 (11.5, -33.24) -> (11.5, -32.24)
  line L547 (11.5, -32.24) -> (12.5, -32.24)
  line L548 (9.5, -32.24) -> (9.5, -33.24)
  line L549 (9.5, -33.24) -> (8.5, -33.24)
  line L550 (8.5, -33.24) -> (8.5, -32.24)
  line L551 (8.5, -32.24) -> (9.5, -32.24)
  line L552 (6.5, -32.24) -> (6.5, -33.24)
  line L553 (6.5, -33.24) -> (5.5, -33.24)
  line L554 (5.5, -33.24) -> (5.5, -32.24)
  line L555 (5.5, -32.24) -> (6.5, -32.24)
  line L556 (3.5, -32.24) -> (3.5, -33.24)
  line L557 (3.5, -33.24) -> (2.5, -33.24)
  line L558 (2.5, -33.24) -> (2.5, -32.24)
  line L559 (2.5, -32.24) -> (3.5, -32.24)
  line L560 (15.5, -34.87) -> (15.5, -35.87)
  line L561 (15.5, -35.87) -> (14.5, -35.87)
  line L562 (14.5, -35.87) -> (14.5, -34.87)
  line L563 (14.5, -34.87) -> (15.5, -34.87)
  line L564 (12.5, -34.87) -> (12.5, -35.87)
  line L565 (12.5, -35.87) -> (11.5, -35.87)
  line L566 (11.5, -35.87) -> (11.5, -34.87)
  line L567 (11.5, -34.87) -> (12.5, -34.87)
  line L568 (9.5, -34.87) -> (9.5, -35.87)
  line L569 (9.5, -35.87) -> (8.5, -35.87)
  line L570 (8.5, -35.87) -> (8.5, -34.87)
  line L571 (8.5, -34.87) -> (9.5, -34.87)
  line L572 (6.5, -34.87) -> (6.5, -35.87)
  line L573 (6.5, -35.87) -> (5.5, -35.87)
  line L574 (5.5, -35.87) -> (5.5, -34.87)
  line L575 (5.5, -34.87) -> (6.5, -34.87)
  line L576 (3.5, -34.87) -> (3.5, -35.87)
  line L577 (3.5, -35.87) -> (2.5, -35.87)
  line L578 (2.5, -35.87) -> (2.5, -34.87)
  line L579 (2.5, -34.87) -> (3.5, -34.87)
  line L580 (15.5, -37.5) -> (15.5, -38.5)
  line L581 (15.5, -38.5) -> (14.5, -38.5)
  line L582 (14.5, -38.5) -> (14.5, -37.5)
  line L583 (14.5, -37.5) -> (15.5, -37.5)
  line L584 (12.5, -37.5) -> (12.5, -38.5)
  line L585 (12.5, -38.5) -> (11.5, -38.5)
  line L586 (11.5, -38.5) -> (11.5, -37.5)
  line L587 (11.5, -37.5) -> (12.5, -37.5)
  line L588 (9.5, -37.5) -> (9.5, -38.5)
  line L589 (9.5, -38.5) -> (8.5, -38.5)
  line L590 (8.5, -38.5) -> (8.5, -37.5)
  line L591 (8.5, -37.5) -> (9.5, -37.5)
  line L592 (6.5, -37.5) -> (6.5, -38.5)
  line L593 (6.5, -38.5) -> (5.5, -38.5)
  line L594 (5.5, -38.5) -> (5.5, -37.5)
  line L595 (5.5, -37.5) -> (6.5, -37.5)
  line L596 (3.5, -37.5) -> (3.5, -38.5)
  line L597 (3.5, -38.5) -> (2.5, -38.5)
  line L598 (2.5, -38.5) -> (2.5, -37.5)
  line L599 (2.5, -37.5) -> (3.5, -37.5)
  line L600 (1, 40.5) -> (1, -40.5)
  line L601 (1, -40.5) -> (26.5, -40.5)
  line L602 (26.5, -40.5) -> (26.5, 40.5)
  line L603 (26.5, 40.5) -> (1, 40.5)
pattern_linear "R-Pattern2" count 30 spacing 2.63 along (0, -1, 0) count 5 spacing 2.8 along (1, 0, 0) of "Extrude4"
sketch "Sketch9" plane through (0, -40.5, 0) normal (0, -1, 0) x (1, 0, 0)
  line L0 (1, 9) -> (1, 5)
  line L1 (1, 5) -> (-1, 5)
  line L2 (-1, 5) -> (-1, 9)
  line L3 (-1, 9) -> (-26.5, 9)
  line L4 (-26.5, 9) -> (-26.5, 0)
  line L5 (-26.5, 0) -> (26.5, 0)
  line L6 (26.5, 0) -> (26.5, 9)
  line L7 (26.5, 9) -> (1, 9)
  line L8 (-20.8174, 4) -> (-23.8174, 4)
  line L9 (-23.8174, 4) -> (-23.8174, -4)
  line L10 (-23.8174, -4) -> (-20.8174, -4)
  line L11 (-20.8174, -4) -> (-20.8174, 4)
  line L12 (-20.8174, 4) -> (-23.8174, -4) construction
  line L13 (-23.8174, 4) -> (-20.8174, -4) construction
  point P0 (-22.3174, 0)
  dimension "d35" = 3
  dimension "d36" = 8
  constraint horizontal L8
  constraint perpendicular L8 L9
  constraint parallel L8 L10
  constraint parallel L9 L11
  constraint coincident L12 P0
  constraint coincident L13 P0
  constraint coincident L5 P0
  measures "d35" distance of L9.end L10.end
  measures "d36" distance of L8.start L10.end
extrude "Extrude6" add sketch "Sketch9" along normal blind 1 contours L5 L8 L9 L11 bodies 1
extrude "Extrude7" add 1 faces at (-21.8174, -41.5, 1.3333) along direction (0, 1, 0) blind 83 on bodies 1 bodies 1
extrude "Extrude8" cut 1 faces at (-21.8174, 41.5, 1.3333) along direction (0, -1, 0) blind 2 on bodies 1 bodies 1
sketch "Sketch10" plane through (0, -40.5, 0) normal (0, -1, 0) x (1, 0, 0)
  line L0 (-20.8174, 4) -> (-20.8174, 0)
  line L1 (-20.8174, 0) -> (26.5, 0)
  line L2 (26.5, 0) -> (26.5, 9)
  line L3 (26.5, 9) -> (1, 9)
  line L4 (1, 9) -> (1, 5)
  line L5 (1, 5) -> (-1, 5)
  line L6 (-1, 5) -> (-1, 9)
  line L7 (-1, 9) -> (-26.5, 9)
  line L8 (-26.5, 9) -> (-26.5, 0)
  line L9 (-26.5, 0) -> (-23.8174, 0)
  line L10 (-23.8174, 0) -> (-23.8174, 4)
  line L11 (-23.8174, 4) -> (-20.8174, 4)
  line L12 (1.5, 4) -> (-1.5, 4)
  line L13 (-1.5, 4) -> (-1.5, -4)
  line L14 (-1.5, -4) -> (1.5, -4)
  line L15 (1.5, -4) -> (1.5, 4)
  line L16 (1.5, 4) -> (-1.5, -4) construction
  line L17 (-1.5, 4) -> (1.5, -4) construction
  dimension "d43" = 3
  dimension "d44" = 8
  constraint horizontal L12
  constraint perpendicular L12 L13
  constraint parallel L12 L14
  constraint parallel L13 L15
  constraint coincident L16 origin
  constraint coincident L17 origin
  measures "d43" distance of L13.end L14.end
  measures "d44" distance of L12.end L13.end
extrude "Extrude9" add sketch "Sketch10" along normal blind 1 contours L1 L12 L13 L15 bodies 1
extrude "Extrude10" add 1 faces at (-0.5, -41.5, 2.6667) along direction (0, 1, 0) blind 83 on bodies 1 bodies 1
extrude "Extrude11" cut 1 faces at (-0.5, 41.5, 2.6667) along direction (0, -1, 0) blind 2 on bodies 1 bodies 1
sketch "Sketch11" plane through (0, -40.5, 0) normal (0, -1, 0) x (1, 0, 0)
  line L0 (1.5, 4) -> (1.5, 0)
  line L1 (1.5, 0) -> (26.5, 0)
  line L2 (26.5, 0) -> (26.5, 9)
  line L3 (26.5, 9) -> (1, 9)
  line L4 (1, 9) -> (1, 5)
  line L5 (1, 5) -> (-1, 5)
  line L6 (-1, 5) -> (-1, 9)
  line L7 (-1, 9) -> (-26.5, 9)
  line L8 (-26.5, 9) -> (-26.5, 0)
  line L9 (-26.5, 0) -> (-23.8174, 0)
  line L10 (-23.8174, 0) -> (-23.8174, 4)
  line L11 (-23.8174, 4) -> (-20.8174, 4)
  line L12 (-20.8174, 4) -> (-20.8174, 0)
  line L13 (-20.8174, 0) -> (-1.5, 0)
  line L14 (-1.5, 0) -> (-1.5, 4)
  line L15 (-1.5, 4) -> (1.5, 4)
  line L16 (24.3656, 4) -> (21.3656, 4)
  line L17 (21.3656, 4) -> (21.3656, -4)
  line L18 (21.3656, -4) -> (24.3656, -4)
  line L19 (24.3656, -4) -> (24.3656, 4)
  line L20 (24.3656, 4) -> (21.3656, -4) construction
  line L21 (21.3656, 4) -> (24.3656, -4) construction
  point P0 (22.8656, 0)
  dimension "d51" = 3
  dimension "d52" = 8
  constraint horizontal L16
  constraint perpendicular L16 L17
  constraint parallel L16 L18
  constraint parallel L17 L19
  constraint coincident L20 P0
  constraint coincident L21 P0
  constraint coincident L1 P0
  measures "d51" distance of L17.end L18.end
  measures "d52" distance of L16.start L18.end
extrude "Extrude12" add sketch "Sketch11" along normal blind 1 contours L1 L16 L17 L19 bodies 1
extrude "Extrude13" add 1 faces at (22.3656, -41.5, 2.6667) along direction (0, 1, 0) blind 83 on bodies 1 bodies 1
extrude "Extrude14" cut 1 faces at (22.3656, 41.5, 2.6667) along direction (0, -1, 0) blind 2 on bodies 1 bodies 1
sketch "Sketch12" plane through (26.5, 0, 0) normal (1, 0, 0) x (0, 1, 0)
  line L0 (-40.5, 0) -> (40.5, 0)
  line L1 (40.5, 0) -> (40.5, 9)
  line L2 (40.5, 9) -> (-40.5, 9)
  line L3 (-40.5, 9) -> (-40.5, 0)
  line L4 (-25.5, -4) -> (-28.5, -4)
  line L5 (-28.5, -4) -> (-28.5, 4)
  line L6 (-28.5, 4) -> (-25.5, 4)
  line L7 (-25.5, 4) -> (-25.5, -4)
  line L8 (-25.5, -4) -> (-28.5, 4) construction
  line L9 (-28.5, -4) -> (-25.5, 4) construction
  point P0 (-27, 0)
  dimension "d59" = 3
  dimension "d60" = 8
  dimension "d76" = 12
  constraint horizontal L4
  constraint perpendicular L4 L5
  constraint parallel L4 L6
  constraint parallel L5 L7
  constraint coincident L8 P0
  constraint coincident L9 P0
  constraint coincident L0 P0
  measures "d59" distance of L5.end L6.end
  measures "d60" distance of L4.start L6.end
  measures "d76" distance of L3 L5
extrude "Extrude15" add sketch "Sketch12" along normal blind 1 contours L0 L5 L6 L7 bodies 1
extrude "Extrude16" add 1 faces at (27.5, -27.5, 2.6667) along direction (-1, 0, 0) blind 55 on bodies 1 bodies 1
extrude "Extrude17" cut 1 faces at (-27.5, -27.5, 2.6667) along direction (1, 0, 0) blind 2 on bodies 1 bodies 1
sketch "Sketch13" plane through (26.5, 0, 0) normal (1, 0, 0) x (0, 1, 0)
  line L0 (-25.5, 4) -> (-25.5, 0)
  line L1 (-25.5, 0) -> (40.5, 0)
  line L2 (40.5, 0) -> (40.5, 9)
  line L3 (40.5, 9) -> (-40.5, 9)
  line L4 (-40.5, 9) -> (-40.5, 0)
  line L5 (-40.5, 0) -> (-28.5, 0)
  line L6 (-28.5, 0) -> (-28.5, 4)
  line L7 (-28.5, 4) -> (-25.5, 4)
  line L8 (28.5, 4) -> (25.5, 4)
  line L9 (25.5, 4) -> (25.5, -4)
  line L10 (25.5, -4) -> (28.5, -4)
  line L11 (28.5, -4) -> (28.5, 4)
  line L12 (28.5, 4) -> (25.5, -4) construction
  line L13 (25.5, 4) -> (28.5, -4) construction
  point P0 (27, 0)
  dimension "d67" = 3
  dimension "d68" = 8
  dimension "d75" = 12
  constraint horizontal L8
  constraint perpendicular L8 L9
  constraint parallel L8 L10
  constraint parallel L9 L11
  constraint coincident L12 P0
  constraint coincident L13 P0
  constraint coincident L1 P0
  measures "d67" distance of L9.end L10.end
  measures "d68" distance of L8.start L10.end
  measures "d75" distance of L2 L11
extrude "Extrude18" add sketch "Sketch13" along normal blind 1 contours L1 L8 L9 L11 bodies 1
extrude "Extrude19" add 1 faces at (27.5, 27.5, 2.6667) along direction (-1, 0, 0) blind 55 on bodies 1 bodies 1
extrude "Extrude20" cut 1 faces at (-27.5, 27.5, 2.6667) along direction (1, 0, 0) blind 2 on bodies 1 bodies 1
sketch "Sketch14" plane through (26.5, 0, 0) normal (1, 0, 0) x (0, 1, 0)
  line L0 (28.5, 4) -> (28.5, 0)
  line L1 (28.5, 0) -> (40.5, 0)
  line L2 (40.5, 0) -> (40.5, 9)
  line L3 (40.5, 9) -> (-40.5, 9)
  line L4 (-40.5, 9) -> (-40.5, 0)
  line L5 (-28.5, 0) -> (-28.5, 4)
  line L6 (-28.5, 4) -> (-25.5, 4)
  line L7 (-25.5, 4) -> (-25.5, 0)
  line L8 (-25.5, 0) -> (25.5, 0)
  line L9 (25.5, 0) -> (25.5, 4)
  line L10 (25.5, 4) -> (28.5, 4)